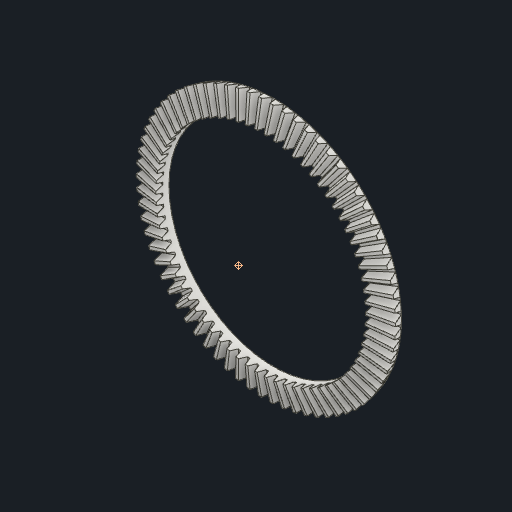
# Autodesk Inventor part: Bevel Gear1
Saved by Autodesk Inventor 2023 (Build 270158000, 158)
## iProperties
CustomPartVersion: 1
Created: 2023-08-11
Part Number: Bevel Gear1
Material: Steel, Mild
Document SubType Name: Modeling
Designer: Izack Waczko
Categories: <?xml version="1.0" encoding="UTF-16"?> <MemberInstance><Categories><FamilyTemplate><FamilyTemplateParameter ValueType="xs:double" Id="1" ObjectReferenceKey="da_z" ObjectType="kUserParameterObject"/><FamilyTemplateParameter ValueType="xs:double" Id="2" ObjectReferenceKey="da_b" ObjectType="kUserParameterObject"/><FamilyTemplateParameter ValueType="xs:double" Id="3" ObjectReferenceKey="da_beta" ObjectType="kUserParameterObject"/><FamilyTemplateParameter ValueType="xs:double" Id="4" ObjectReferenceKey="da_dae" ObjectType="kUserParameterObject"/><FamilyTemplateParameter ValueType="xs:double" Id="5" ObjectReferenceKey="da_ve" ObjectType="kUserParameterObject"/><FamilyTemplateParameter ValueType="xs:double" Id="6" ObjectReferenceKey="da_omega" ObjectType="kUserParameterObject"/><FamilyTemplateParameter ValueType="xs:string" Id="7" ObjectReferenceKey="EAIAABAAAAAAHwAAAAAAAIAAAAAAAAAA" ObjectType="83914240" SubObjectId="SurfaceGeometry"/></FamilyTemplate><ParamToTemplateMap><ParamToTemplate CategoryParameter="//CategoryParameter[@InternalName='046C89C9-8512-4d59-83FE-43B91F4F132A']" TemplateParameter="1"/><ParamToTemplate CategoryParameter="//CategoryParameter[@InternalName='2552DF32-E462-4b46-AEBF-C6C7768E72AC']" TemplateParameter="2"/><ParamToTemplate CategoryParameter="//CategoryParameter[@InternalName='C9EE641D-15FC-4fae-A226-E94C4372FDD7']" TemplateParameter="3"/><ParamToTemplate><ParamToTemplate CategoryParameter="//CategoryParameter[@InternalName='00B6519A-459B-49c7-AD84-2E56D39A5744']" ConstantValue="0.000000"/></ParamToTemplate><ParamToTemplate><ParamToTemplate CategoryParameter="//CategoryParameter[@InternalName='04B31F0E-C7A6-4894-AA32-9629BEFACF47']" ConstantValue="1.000000"/></ParamToTemplate><ParamToTemplate><ParamToTemplate CategoryParameter="//CategoryParameter[@InternalName='43CBEC2E-7847-49e7-A936-2F7889FCB2D9']" ConstantValue="0.200000"/></ParamToTemplate><ParamToTemplate><ParamToTemplate CategoryParameter="//CategoryParameter[@InternalName='B1EFC894-105D-4ebd-86BF-FA20ED196853']" ConstantValue="0.300000"/></ParamToTemplate><ParamToTemplate><ParamToTemplate CategoryParameter="//CategoryParameter[@InternalName='51175063-3D10-4879-93E8-6246FE8B403D']" ConstantValue="2060000000.000000"/></ParamToTemplate><ParamToTemplate><ParamToTemplate CategoryParameter="//CategoryParameter[@InternalName='A3A52E27-4454-46a9-B0BD-C932399B70AF']" ConstantValue="0.300000"/></ParamToTemplate><ParamToTemplate CategoryParameter="//CategoryParameter[@InternalName='2A200944-5A8C-41ca-B96E-8520D2E510F1']" TemplateParameter="4"/><ParamToTemplate><ParamToTemplate CategoryParameter="//CategoryParameter[@InternalName='1A637F62-92C8-44bc-B81F-10802510B579']" ConstantValue="5.677571"/></ParamToTemplate><ParamToTemplate CategoryParameter="//CategoryParameter[@InternalName='B52DD4BE-6863-48fb-BF58-89EF6F9EC65C']" TemplateParameter="5"/><ParamToTemplate><ParamToTemplate CategoryParameter="//CategoryParameter[@InternalName='3956BFF2-84D2-457d-93C2-9B0613DEBA67']" ConstantValue="0.606513"/></ParamToTemplate><ParamToTemplate CategoryParameter="//CategoryParameter[@InternalName='739CFA02-461B-4bf8-8049-181FCAD8B28F']" TemplateParameter="6"/><ParamToTemplate><ParamToTemplate CategoryParameter="//CategoryParameter[@InternalName='A27E999F-E2CE-4481-8A2A-EBF499C4C3C5']" ConstantValue="0.000000"/></ParamToTemplate><ParamToTemplate><ParamToTemplate CategoryParameter="//CategoryParameter[@InternalName='9E1B4470-B2D3-4ff1-B813-535BB4CDF51A']" ConstantValue="3520000.000000"/></ParamToTemplate><ParamToTemplate><ParamToTemplate CategoryParameter="//CategoryParameter[@InternalName='F8452263-BFF6-458c-9FB1-07C4B99E95CD']" ConstantValue="11400000.000000"/></ParamToTemplate><ParamToTemplate><ParamToTemplate CategoryParameter="//CategoryParameter[@InternalName='3E3BB259-FD49-497f-8171-6EBC954A3479']" ConstantValue="2.000000"/></ParamToTemplate><ParamToTemplate CategoryParameter="//CategoryParameter[@InternalName='27C3BAF2-7550-4e4b-AE2C-0DB134B7D9B7']" TemplateParameter="7"/></ParamToTemplateMap><Category DisplayName="Gear" InternalName="DC85795E-93AB-48d5-8EEE-5A27447B64BD" Mnemonic="Gear"><CategoryParameter DisplayName="z" InternalName="046C89C9-8512-4d59-83FE-43B91F4F132A" Mnemonic="z"/><CategoryParameter DisplayName="b" InternalName="2552DF32-E462-4b46-AEBF-C6C7768E72AC" Mnemonic="b"/><CategoryParameter DisplayName="||b|" InternalName="C9EE641D-15FC-4fae-A226-E94C4372FDD7" Mnemonic="beta"/><CategoryParameter DisplayName="x" InternalName="00B6519A-459B-49c7-AD84-2E56D39A5744" Mnemonic="x"/><CategoryParameter DisplayName="a*" InternalName="04B31F0E-C7A6-4894-AA32-9629BEFACF47" Mnemonic="a"/><CategoryParameter DisplayName="c*" InternalName="43CBEC2E-7847-49e7-A936-2F7889FCB2D9" Mnemonic="c"/><CategoryParameter DisplayName="r|.f|*" InternalName="B1EFC894-105D-4ebd-86BF-FA20ED196853" Mnemonic="rf"/><CategoryParameter DisplayName="E" InternalName="51175063-3D10-4879-93E8-6246FE8B403D" Mnemonic="E"/><CategoryParameter DisplayName="||m|" InternalName="A3A52E27-4454-46a9-B0BD-C932399B70AF" Mnemonic="mi"/><Category DisplayName="BevelGear" InternalName="0C98F69A-0C2B-4791-B2FE-7691BB227E77" Mnemonic="BevelGear"><CategoryParameter DisplayName="d|.ae|" InternalName="2A200944-5A8C-41ca-B96E-8520D2E510F1" Mnemonic="dae"/><CategoryParameter DisplayName="d|.ai|" InternalName="1A637F62-92C8-44bc-B81F-10802510B579" Mnemonic="dai"/><CategoryParameter DisplayName="A|.e|" InternalName="B52DD4BE-6863-48fb-BF58-89EF6F9EC65C" Mnemonic="ve"/><CategoryParameter DisplayName="A|.i|" InternalName="3956BFF2-84D2-457d-93C2-9B0613DEBA67" Mnemonic="vi"/><CategoryParameter DisplayName="||S|" InternalName="739CFA02-461B-4bf8-8049-181FCAD8B28F" Mnemonic="omega"/><CategoryParameter DisplayName="x|.t|" InternalName="A27E999F-E2CE-4481-8A2A-EBF499C4C3C5" Mnemonic="xt"/><CategoryParameter DisplayName="||s||.Flim|" InternalName="9E1B4470-B2D3-4ff1-B813-535BB4CDF51A" Mnemonic="sFlim"/><CategoryParameter DisplayName="||s||.Hlim|" InternalName="F8452263-BFF6-458c-9FB1-07C4B99E95CD" Mnemonic="sHlim"/><CategoryParameter DisplayName="type" InternalName="3E3BB259-FD49-497f-8171-6EBC954A3479" Mnemonic="type"/><CategoryParameter DisplayName="PitchDiameter" InternalName="27C3BAF2-7550-4e4b-AE2C-0DB134B7D9B7" Mnemonic="IDS_PITCHDIAM"/></Category></Category></Categories></MemberInstance>
Mass: 60.9118 g
Surface Area: 34.3074 cm^2
Volume: 7.7496 cm^3
Density: 7.86 g/cm^3
Appearance: Steel
Author: Izack Waczko
Autodesk Inventor part; units mm, degrees
ref_plane "Mesh Plane2" through (0, 0, 0) normal (0.9989931, 0.0448648, 0) x (0, 0, 1)
sketch "Teeth Body Sketch" plane through (0, 0, 0) normal (1, 0, 0) x (0, 1, 0)
  line L0 (0, 0) -> (34.7168, -9.6661) construction
  line L1 (34.7168, -9.6661) -> (35.236, -7.5282)
  line L2 (35.236, -7.5282) -> (0, 0) construction
  line L3 (35, -8.5) -> (0, 0) construction
  line L4 (27.9696, -7.7875) -> (28.3879, -6.0651)
  line L5 (34.7168, -9.6661) -> (27.9696, -7.7875)
  line L6 (35.236, -7.5282) -> (28.3879, -6.0651)
  line L7 (0, -11.597) -> (0, 1.9328) projected
  line L8 (0, -8.5) -> (35.236, -8.5) construction
  dimension "d0" = 70
  dimension "d1" = 69.4336
  dimension "d2" = 70.472
  dimension "d3" = 7
  dimension "d4" = 7.5282
  constraints: 16 end point, 4 point on line, 3 perpendicular, 2 collinear, 1 horizontal alignment, 1 vertical alignment
  measures "d0" diameter of L3.start L7
  measures "d1" diameter of L0.end L7
  measures "d2" diameter of L1.end L7
  measures "d3" distance between parallel lines of L1 L4
  measures "d4" vertical distance of L1.end L0.start
revolve "Teeth Body" add sketch "Teeth Body Sketch" angle 360 about axis through (0, 0, 0) along (0, 0, 1)
ref_plane "Tooth Plane" through (0, 35, -8.5) normal (0, -0.9717537, 0.2359973) x (1, 0, 0)
sketch "Start Sketch" plane through (0, 35, -8.5) normal (0, -0.9717537, 0.2359973) x (1, 0, 0)
  line L0 (0, -168.5552) -> (0, 30.0321) projected
  arc A0 (-0.303, -1.464) -> (-1.4106, 1.6534) centre (-48.958, -16.9951) ccw
  arc A1 (1.4106, 1.6534) -> (0.303, -1.464) centre (48.958, -16.9951) ccw
  line L1 (-0.303, -1.464) -> (0.303, -1.464)
  arc A2 (1.4106, 1.6534) -> (-1.4106, 1.6534) centre (0, -148.3068) ccw
  dimension "d7" = 51.0737
  dimension "d8" = 48.958
  dimension "d9" = 131.3116
  dimension "d57" = 149.9668
  dimension "d58" = 146.8428
  constraints: 6 point on circle, 3 centre point, 3 symmetric about line, 2 end point, 1 coincident, 1 perpendicular, 1 other
  measures "d7" radius of A0
  measures "d8" horizontal distance of point (0, -148.307) A0.centre
  measures "d9" vertical distance of point (0, -148.307) A0.centre
  measures "d57" radius of A2
  measures "d58" distance from line of A2.centre L1
sketch "End Sketch" plane through (0, 28.0908, -6.8221) normal (0, -0.9717537, 0.2359973) x (1, 0, 0)
  line L0 (0, -134.3597) -> (0, 23.9393) projected
  arc A0 (-0.2432, -1.175) -> (-1.1321, 1.327) centre (-39.2935, -13.6402) ccw
  arc A1 (1.1321, 1.327) -> (0.2432, -1.175) centre (39.2935, -13.6402) ccw
  line L1 (-0.2432, -1.175) -> (0.2432, -1.175)
  arc A2 (1.1321, 1.327) -> (-1.1321, 1.327) centre (0, -119.0303) ccw
  dimension "d12" = 40.9915
  dimension "d15" = 39.2935
  dimension "d16" = 105.3901
  dimension "d59" = 120.3626
  dimension "d60" = 117.8553
  constraints: 6 point on circle, 3 centre point, 3 symmetric about line, 2 end point, 1 coincident, 1 other
  measures "d12" radius of A0
  measures "d15" horizontal distance of A0.centre point (0, -119.03)
  measures "d16" vertical distance of A0.centre point (0, -119.03)
  measures "d59" radius of A2
  measures "d60" distance from line of A2.centre L1
loft "Loft" cut profiles "Start Sketch", "End Sketch"
pattern_circular "Circular Pattern" count 70 over 360 about axis through (0, 0, 0) along (0, 0, 1) of "Loft"
ref_plane "End Plane" through (0, 28.0908, -6.8221) normal (0, -0.9717537, 0.2359973) x (1, 0, 0)
sketch3d "3D Sketch Right"
ref_plane "End Plane Right" through (-2.6548, 27.9651, -6.8221) normal (0.0918374, -0.9674043, 0.2359973) x (0.9955242, 0.0945068, 0)
sketch "End Sketch Right" plane through (-2.6548, 27.9651, -6.8221) normal (0.0918374, -0.9674043, 0.2359973) x (0.9955242, 0.0945068, 0)
  arc A0 (-0.2432, -1.175) -> (-1.1321, 1.327) centre (-39.2935, -13.6402) ccw
  line L0 (0, -145.3975) -> (0, 27.6924) projected
  arc A1 (1.1321, 1.327) -> (0.2432, -1.175) centre (39.2935, -13.6402) ccw
  line L1 (-0.2432, -1.175) -> (0.2432, -1.175)
  arc A2 (1.1321, 1.327) -> (-1.1321, 1.327) centre (0, -119.0303) ccw
  dimension "d70" = 39.2935
  dimension "d71" = 105.3901
  dimension "d72" = 40.9915
  dimension "d73" = 117.8553
  dimension "d74" = 120.3626
  constraints: 6 point on circle, 3 centre point, 3 symmetric about line, 2 end point, 1 coincident, 1 perpendicular, 1 other
  measures "d70" horizontal distance of A2.centre A0.centre
  measures "d71" vertical distance of point (0, -119.03) A0.centre
  measures "d72" radius of A0
  measures "d73" distance from line of point (0, -119.03) L1
  measures "d74" radius of A2
feature "Loft Right" [suppressed]
pattern_circular "Circular Pattern Right" [suppressed]
sketch3d "3D Sketch Left"
ref_plane "End Plane Left" through (2.7116, 27.9651, -6.9155) normal (-0.0937131, -0.9664863, 0.2390021) x (0.995332, -0.0965101, 0)
sketch "End Sketch Left" plane through (2.7116, 27.9651, -6.9155) normal (-0.0937131, -0.9664863, 0.2390021) x (0.995332, -0.0965101, 0)
  line L0 (0, -145.385) -> (0, 27.8575) projected
  arc A0 (-0.2432, -1.085) -> (-1.1321, 1.417) centre (-39.2935, -13.5502) ccw
  arc A1 (1.1321, 1.417) -> (0.2432, -1.085) centre (39.2935, -13.5502) ccw
  line L1 (-0.2432, -1.085) -> (0.2432, -1.085)
  ellipse E0 centre (0, -5.8894) end of major axis (28.3879, -5.8894) minor radius 6.7848 projected
  arc A2 (1.1321, 1.417) -> (-1.1321, 1.417) centre (0, -118.9403) ccw
  dimension "d56" = 6.7848
  dimension "d30" = 40.9915
  dimension "d31" = 39.2935
  dimension "d32" = 105.3901
  dimension "d61" = 120.3626
  dimension "d62" = 117.8553
  constraints: 6 point on circle, 3 centre point, 3 symmetric about line, 2 end point, 1 coincident, 2 other
  measures "d30" radius of A0
  measures "d31" horizontal distance of point (0, -118.94) A0.centre
  measures "d32" vertical distance of A0.centre point (0, -118.94)
  measures "d61" radius of A2
  measures "d62" distance from line of point (0, -118.94) L1
feature "Loft Left" [suppressed]
pattern_circular "Circular Pattern Left" [suppressed]
sketch "Body Sketch" plane through (0, 0, 0) normal (1, 0, 0) x (0, 1, 0)
  line L0 (0, -10.0502) -> (0, -7.3478) projected
  line L1 (34.7168, -9.6661) -> (27.9696, -7.7875) projected
  line L2 (27.9696, -7.7875) -> (0, -7.7875)
  line L3 (34.7168, -9.6661) -> (0, -9.6661)
  constraints: 4 end point, 2 perpendicular, 2 point on line
revolve "Fix Body" add sketch "Body Sketch" angle 360 about axis through (0, 0, 0) along (0, 0, 1)
sketch "Sketch6" plane through (0, 0, 0) normal (1, 0, 0) x (0, 1, 0)
  line L0 (35, -8.5) -> (0, 0) projected
  line L1 (0, -10.2) -> (0, 1.7) projected
surface revolve "Pitch Diameter" sketch "Sketch6" angle 360 about axis through (0, 0, 0) along (0, 0, 1) shown no curves L0
sketch "Sketch8" plane through (0, 0, -9.6661) normal (0, 0, -1) x (-1, 0, 0)
  circle A0 centre (0, 0) radius 28.5
  dimension "d94" = 57
  constraints: 1 centre point, 1 coincident
  measures "d94" diameter of A0
extrude "Extrusion1" cut sketch "Sketch8" against normal blind 10
equation "\"d0\" = da_de"
equation "\"d1\" = da_dfe"
equation "\"d2\" = da_dae"
equation "\"d3\" = da_b"
equation "\"d4\" = da_ve"
equation "\"d7\" = fd_rr"
equation "\"d8\" = fd_x"
equation "\"d9\" = fd_y"
equation "\"d57\" = 0.5 * fd_dva + 0.3 * da_he"
equation "\"d58\" = 0.5 * fd_dva - 1.12 * da_he"
equation "\"da_teethtype\" = 0"
equation "\"da_b\" = 7"
equation "\"da_de\" = 70"
equation "\"da_dae\" = 70.47199"
equation "\"da_dfe\" = 69.43361"
equation "\"da_le\" = 36.01736"
equation "\"da_omega\" = 90deg"
equation "\"da_beta\" = 0"
equation "\"da_delta\" = 76.349581deg"
equation "\"da_alpha\" = 20deg"
equation "\"da_he\" = 2.2"
equation "\"da_ve\" = 7.52825"
equation "\"da_zv\" = 296.613528"
equation "\"fd_loft\" = da_b + 0.05 * da_he"
equation "\"fd_x\" = fd_x1 + fd_x2"
equation "\"fd_y\" = fd_y1 - fd_y2"
equation "\"fd_dd\" = fd_dva - 0.8 * da_he"
equation "\"da_dvw\" = 296.61353"
equation "\"d11\" = fd_loft"
equation "\"da_dm\" = 63.19772"
equation "\"da_x\" = 0"
equation "\"da_m\" = 1"
equation "\"d50\" = da_omega"
equation "\"fd_rr\" = 51.073693"
equation "\"fd_dva\" = 298.613528"
equation "\"fd_x1\" = 0.794121"
equation "\"fd_x2\" = 48.163884"
equation "\"fd_y1\" = 148.304638"
equation "\"fd_y2\" = 16.993011"
body "Solid1"
body "Srf1"
